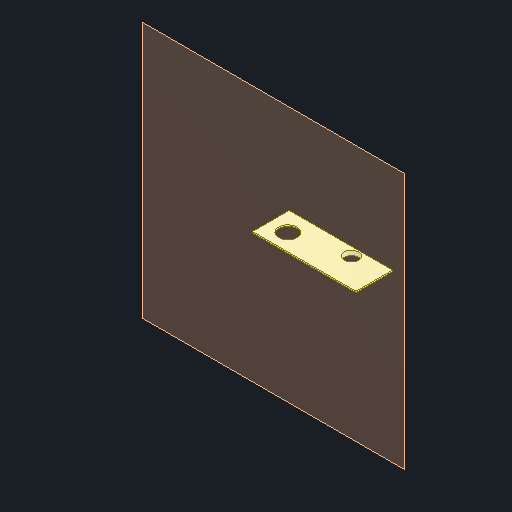
# Autodesk Inventor part: right_hold
Saved by Autodesk Inventor 2023 (Build 270158000, 158)
## iProperties
Created: 2024-05-18
Part Number: right_hold
Material: Nylon 6/6
Document SubType Name: Modeling
Designer: szymo
Density: 1.13 g/cm^3
Appearance: Nylon 6
Mass: 2.55547 g
Surface Area: 45.3771 cm^2
Volume: 2.26148 cm^3
Author: szymo
Autodesk Inventor part; units mm, degrees
ref_plane "YZ Plane" through (0, 0, 0) normal (1, 0, 0) x (0, 1, 0)
ref_plane "XZ Plane" through (0, 0, 0) normal (0, 1, 0) x (-1, 0, 0)
ref_plane "XY Plane" through (0, 0, 0) normal (0, 0, 1) x (1, 0, 0)
ref_plane "Work Plane1" through (0, 0, 0) normal (0, 0, 1) x (1, 0, 0)
sketch "Sketch1" plane through (0, 0, 0) normal (0, 0, 1) x (1, 0, 0)
  line L0 (-71, -74) -> (-71, -89) projected
  line L1 (-71, -89) -> (41, -89) projected
  line L2 (41, -89) -> (41, -30.5) projected
  line L3 (41, -30.5) -> (91, -30.5) projected
  line L4 (91, -30.5) -> (91, 30.5) projected
  line L5 (91, 30.5) -> (41, 30.5) projected
  line L6 (41, 30.5) -> (41, 89) projected
  line L7 (41, 89) -> (-71, 89) projected
  line L8 (-71, 89) -> (-71, 74) projected
  line L9 (-71, 74) -> (-87, 74) projected
  line L10 (-87, 74) -> (-87, 89) projected
  line L11 (-87, 89) -> (-91, 89) projected
  line L12 (-91, 89) -> (-91, -89) projected
  line L13 (-91, -89) -> (-87, -89) projected
  line L14 (-87, -89) -> (-87, -74) projected
  line L15 (-87, -74) -> (-71, -74) projected
  line L16 (91, 29.5) -> (12, 29.5)
  line L17 (12, 29.5) -> (12, 28.5)
  line L18 (12, 28.5) -> (91, 28.5)
  line L19 (91, 28.5) -> (91, 29.5)
  line L20 (71.5, 26) -> (60.5, 26) projected
  line L21 (12, 37) -> (40, 37) projected
  line L22 (11, 8.5) -> (11, 9.5)
  point P0 (0, 0)
  dimension "d0" = 1
  dimension "d1" = 2.5
  dimension "d2" = 1
  dimension "d14" = 1
  constraints: 10 end point, 2 parallel, 1 horizontal, 1 perpendicular, 1 point on line, 1 vertical, 2 other
  measures "d0" distance between parallel lines of L5 L16
  measures "d1" distance between parallel lines of L18 L20
  measures "d2" distance between parallel lines of L16 L18
  measures "d14" distance between parallel lines of L22 L17
ref_plane "Work Plane2" through (11, 8.5, 30) normal (0, 0, 1) x (1, 0, 0)
extrude "Extrusion1" add sketch "Sketch1" along normal blind 28 contours L18 L17 L16 L4
sketch "Sketch2" plane through (12, 28.5, 0) normal (0, -1, 0) x (1, 0, 0)
  circle A0 centre (54, 6.5) radius 5.5 projected
  arc A1 (11.5575, 17.9943) -> (9.6437, 18.8944) centre (8.6132, 14.2185) ccw projected
  arc A2 (9.6437, 18.8944) -> (9.0881, 18.165) centre (14, 15) ccw projected
  arc A3 (9.0881, 18.165) -> (10.4644, 16.5591) centre (13.322, 20.4008) ccw projected
  arc A4 (10.4644, 16.5591) -> (10.264, 15.9868) centre (14, 15) ccw projected
  arc A5 (10.264, 15.9868) -> (8.1866, 15.59) centre (10.1013, 11.2015) ccw projected
  arc A6 (8.1866, 15.59) -> (8.1659, 14.6734) centre (14, 15) ccw projected
  arc A7 (8.1659, 14.6734) -> (10.2232, 14.1831) centre (10.277, 18.9709) ccw projected
  arc A8 (10.2232, 14.1831) -> (10.3975, 13.6024) centre (14, 15) ccw projected
  arc A9 (10.3975, 13.6024) -> (8.95, 12.0603) centre (13.0786, 9.6353) ccw projected
  arc A10 (8.95, 12.0603) -> (9.4721, 11.3065) centre (14, 15) ccw projected
  arc A11 (9.4721, 11.3065) -> (11.4247, 12.1192) centre (8.654, 16.0242) ccw projected
  arc A12 (11.4247, 12.1192) -> (11.907, 11.7518) centre (14, 15) ccw projected
  arc A13 (11.907, 11.7518) -> (11.6424, 9.6535) centre (16.4078, 10.1183) ccw projected
  arc A14 (11.6424, 9.6535) -> (12.5078, 9.3505) centre (14, 15) ccw projected
  arc A15 (12.5078, 9.3505) -> (13.6098, 11.1556) centre (9.073, 12.6863) ccw projected
  arc A16 (13.6098, 11.1556) -> (14.216, 11.1419) centre (14, 15) ccw projected
  arc A17 (14.216, 11.1419) -> (15.2353, 9.2888) centre (18.8174, 12.4659) ccw projected
  arc A18 (15.2353, 9.2888) -> (16.1135, 9.5523) centre (14, 15) ccw projected
  arc A19 (16.1135, 9.5523) -> (15.944, 11.6605) centre (11.3739, 10.2321) ccw projected
  arc A20 (15.944, 11.6605) -> (16.4425, 12.0057) centre (14, 15) ccw projected
  arc A21 (16.4425, 12.0057) -> (18.3563, 11.1056) centre (19.3868, 15.7815) ccw projected
  arc A22 (18.3563, 11.1056) -> (18.9119, 11.835) centre (14, 15) ccw projected
  arc A23 (18.9119, 11.835) -> (17.5356, 13.4409) centre (14.678, 9.5992) ccw projected
  arc A24 (17.5356, 13.4409) -> (17.736, 14.0132) centre (14, 15) ccw projected
  arc A25 (17.736, 14.0132) -> (19.8134, 14.41) centre (17.8987, 18.7985) ccw projected
  arc A26 (19.8134, 14.41) -> (19.8341, 15.3266) centre (14, 15) ccw projected
  arc A27 (19.8341, 15.3266) -> (17.7768, 15.8169) centre (17.723, 11.0291) ccw projected
  arc A28 (17.7768, 15.8169) -> (17.6025, 16.3976) centre (14, 15) ccw projected
  arc A29 (17.6025, 16.3976) -> (19.05, 17.9397) centre (14.9214, 20.3647) ccw projected
  arc A30 (19.05, 17.9397) -> (18.5279, 18.6935) centre (14, 15) ccw projected
  arc A31 (18.5279, 18.6935) -> (16.5753, 17.8808) centre (19.346, 13.9758) ccw projected
  arc A32 (16.5753, 17.8808) -> (16.093, 18.2482) centre (14, 15) ccw projected
  arc A33 (16.093, 18.2482) -> (16.3576, 20.3465) centre (11.5922, 19.8817) ccw projected
  arc A34 (16.3576, 20.3465) -> (15.4922, 20.6495) centre (14, 15) ccw projected
  arc A35 (15.4922, 20.6495) -> (14.3902, 18.8444) centre (18.927, 17.3137) ccw projected
  arc A36 (14.3902, 18.8444) -> (13.784, 18.8581) centre (14, 15) ccw projected
  arc A37 (13.784, 18.8581) -> (12.7647, 20.7112) centre (9.1826, 17.5341) ccw projected
  arc A38 (12.7647, 20.7112) -> (11.8865, 20.4477) centre (14, 15) ccw projected
  arc A39 (11.8865, 20.4477) -> (12.056, 18.3395) centre (16.6261, 19.7679) ccw projected
  arc A40 (12.056, 18.3395) -> (11.5575, 17.9943) centre (14, 15) ccw projected
  circle A41 centre (14, 15) radius 5.8433
  circle A42 centre (14, 15) radius 7
  point P0 (-12, 0)
  dimension "d12" = 11.6865
  dimension "d13" = 14
  constraints: 2 centre point, 2 coincident
  measures "d12" diameter of A41
  measures "d13" diameter of A42
extrude "Extrusion2" cut sketch "Sketch2" against normal up to next contours A0 | A40 A39 A38 A37 A36 A35 A34 A33 A32 A31 A30 A29 A28 A27 A26 A25 A24 A23 A22 A21 A20 A19 A18 A17 A16 A15 A14 A13 A12 A11 A10 A9 A8 A7 A6 A5 A4 A3 A2 A1 | A1 A41 A39 A40 | A3 A4 A5 A41 | A41 A35 A36 A37 | A7 A8 A9 A41 | A41 A31 A32 A33 | A11 A12 A13 A41 | A41 A27 A28 A29 | A15 A16 A17 A41 | A19 A20 A21 A41 | A41 A23 A24 A25 | A42
sketch "Sketch3" plane through (12, 28.5, 0) normal (0, -1, 0) x (1, 0, 0)
  circle A0 centre (24.2408, 2.7067) radius 2 projected
  circle A1 centre (54, 6.5) radius 5.5 projected
  circle A2 centre (54, 6.5) radius 7.5
  circle A3 centre (24.2408, 2.7067) radius 4
  point P0 (-12, 0)
  dimension "d8" = 2
  dimension "d9" = 2
  constraints: 2 centre point
  measures "d8" radial gap between concentric circles of A1 A2
  measures "d9" radial gap between concentric circles of A0 A3
ref_plane "Work Plane3" through (58.3168, 26, -1.1832) normal (0, -1, 0) x (0.8086551, 0, -0.588283)
extrude "Extrusion3" add sketch "Sketch3" along normal up to surface (2.5 mm away)
body "Solid1"
